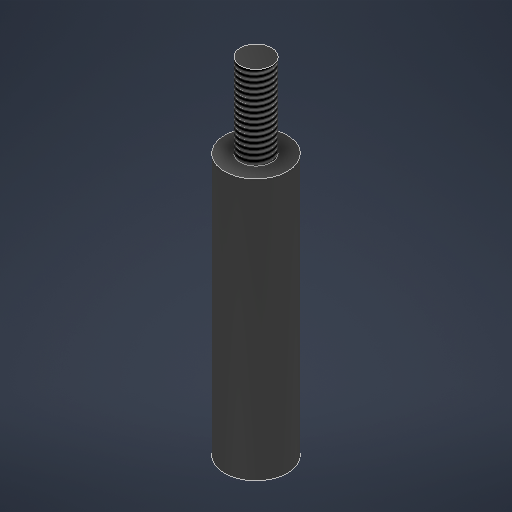
# Autodesk Inventor part: Abstandsbolzen PA6.6 schwarz IA Ø6x20 I=M3x10 A=M3x8 o. Freistich
Saved by Autodesk Inventor 2026.1 (Build 301233020, 233B)
## iProperties
Created: 2026-04-17
Part Number: Abstandsbolzen PA6.6 schwarz IA Ø6x20 I=M3x10 A=M3x8 o. Freistich
Material: Generic
Document SubType Name: Modeling
Designer: Bahaa
Mass: 0.692721 g
Surface Area: 6.97434 cm^2
Volume: 0.692721 cm^3
Density: 1 g/cm^3
Appearance: Glossy - Black
Author: Bahaa
Autodesk Inventor part; units mm, degrees
ref_plane "YZ Plane" through (0, 0, 0) normal (1, 0, 0) x (0, 1, 0)
ref_plane "XZ Plane" through (0, 0, 0) normal (0, 1, 0) x (-1, 0, 0)
ref_plane "XY Plane" through (0, 0, 0) normal (0, 0, 1) x (1, 0, 0)
sketch "Sketch1" plane through (0, 0, 0) normal (0, 0, 1) x (1, 0, 0)
  circle A0 centre (0, 0) radius 3
  circle A1 centre (0, 0) radius 1.5
  dimension "d0" = 6
  dimension "d1" = 3
  constraints: 2 centre point, 2 coincident
  measures "d0" diameter of A0
  measures "d1" diameter of A1
extrude "Extrusion1" add sketch "Sketch1" along normal blind 25 contours A0 | A1
extrude "Extrusion2" cut sketch "Sketch1" along normal blind 10 contours A1
extrude "Extrusion3" add sketch "Sketch1" along normal blind 8 from surface at 25 contours A1
thread "Thread1" size "M3x0.5" class "6g" standard "ANSI Metric M Profile" full length
thread "Thread2" size "M3x0.5" class "6H" standard "ANSI Metric M Profile" full length
body "Solid1"
